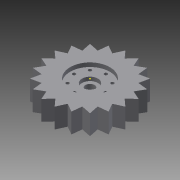
# Autodesk Inventor part: JointSmallGear
Saved by Autodesk Inventor 2015 (Build 190159000, 159)
## iProperties
Created: 2016-04-10
Part Number: JointSmallGear
Material: Generic
Document SubType Name: Modeling
Designer: Hatch
Density: 1 g/cm^3
Appearance: Default
Author: Hatch
Autodesk Inventor part; units mm, degrees
ref_plane "YZ Plane" through (0, 0, 0) normal (1, 0, 0) x (0, 1, 0)
ref_plane "XZ Plane" through (0, 0, 0) normal (0, 1, 0) x (-1, 0, 0)
ref_plane "XY Plane" through (0, 0, 0) normal (0, 0, 1) x (1, 0, 0)
sketch "Sketch1" plane through (0, 0, 0) normal (0, 1, 0) x (-1, 0, 0)
  circle A0 centre (0, 0) radius 17.5
  dimension "d0" = 35
  constraints: 1 centre point, 1 coincident
  measures "d0" diameter of A0
extrude "Base" add sketch "Sketch1" along normal blind 10
sketch "Sketch2" plane through (0, 10, 0) normal (0, 1, 0) x (1, 0, 0)
  circle A0 centre (0, 0) radius 8
  circle A1 centre (-8, 0) radius 0.8
  dimension "d3" = 16
  dimension "d4" = 1.6
  constraints: 1 centre point, 1 coincident, 1 horizontal alignment, 2 other
  measures "d4" diameter of A1
extrude "Mounting Hole" cut sketch "Sketch2" against normal through all contours A1 A0 | A0 A1 picked at (-7.7304, 0) picked at (-8.2616, 0.0332)
pattern_circular "Circular Pattern1" count 8 over 360 about axis through (0, 0, 0) along (0, 1, 0) of "Mounting Hole"
sketch "Sketch3" plane through (0, 10, 0) normal (0, 1, 0) x (1, 0, 0)
  arc A0 (-16.6435, 5.4078) -> (-17.5, 0) centre (0, 0) ccw
  line L0 (0, 0) -> (-16.6435, 5.4078) construction
  line L1 (0, 0) -> (-17.5, 0) construction
  line L2 (0, 0) -> (-25.2614, 4.001)
  line L3 (0, 0) -> (25.5763, 0) construction
  line L4 (-17.5, 0) -> (-21.2042, 3.3584)
  line L5 (-16.6435, 5.4078) -> (-21.2042, 3.3584)
  dimension "d11" = 18
  dimension "d12" = 171
  dimension "d13" = 5
  constraints: 12 end point, 2 point on circle, 1 centre point, 1 coincident, 1 equal length, 1 horizontal, 1 point on line
  measures "d11" angle of L0 L1
  measures "d12" angle of L3 L2
  measures "d13" distance of L1.end L4.end
extrude "Gear Tooth" add sketch "Sketch3" against normal blind 10
pattern_circular "Circular Pattern2" count 20 over 360 about axis through (0, 0, 0) along (0, 1, 0) of "Gear Tooth"
sketch "Sketch6" plane through (0, 10, 0) normal (0, 1, 0) x (1, 0, 0)
  point P0 (0, 0)
sketch "Sketch7" plane through (0, 10, 0) normal (0, 1, 0) x (1, 0, 0)
  circle A0 centre (0, 0) radius 10
  dimension "d26" = 20
  constraints: 1 centre point, 1 coincident
  measures "d26" diameter of A0
extrude "Extrusion6" cut sketch "Sketch7" against normal blind 2
sketch "Sketch8" plane through (0, 8, 0) normal (0, 1, 0) x (1, 0, 0)
  circle A0 centre (0, 0) radius 4
  dimension "d29" = 8
  constraints: 1 centre point, 1 coincident
  measures "d29" diameter of A0
extrude "Extrusion7" cut sketch "Sketch8" against normal blind 1.9
sketch "Sketch9" plane through (0, 6.1, 0) normal (0, 1, 0) x (1, 0, 0)
  circle A0 centre (0, 0) radius 2.25
  dimension "d32" = 4.5
  constraints: 1 centre point, 1 coincident
  measures "d32" diameter of A0
extrude "Extrusion8" cut sketch "Sketch9" against normal blind 2.5
body "Solid1"
